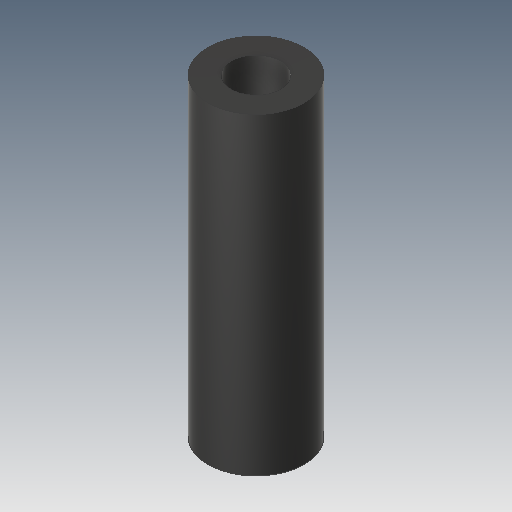
# Autodesk Inventor part: 20mm Nylon Stand Off
Saved by Autodesk Inventor 2019 (Build 230136000, 136)
## iProperties
Created: 2018-10-05
Part Number: 20mm Nylon Stand Off
Material: Acetal Resin, Black
Document SubType Name: Modeling
Designer: Ax
Density: 1.425 g/cm^3
Appearance: Smooth - Black
Mass: 0.637537 g
Surface Area: 6.40822 cm^2
Volume: 0.447394 cm^3
Author: Ax
Autodesk Inventor part; units mm, degrees
ref_plane "YZ Plane" through (0, 0, 0) normal (1, 0, 0) x (0, 1, 0)
ref_plane "XZ Plane" through (0, 0, 0) normal (0, 1, 0) x (-1, 0, 0)
ref_plane "XY Plane" through (0, 0, 0) normal (0, 0, 1) x (1, 0, 0)
sketch "Sketch1" plane through (0, 0, 0) normal (0, 1, 0) x (-1, 0, 0)
  circle A0 centre (0, 0) radius 3.1
  circle A1 centre (0, 0) radius 1.6
  dimension "d0" = 6.2
  dimension "d1" = 3.2
  constraints: 2 centre point, 2 coincident
  measures "d0" diameter of A0
  measures "d1" diameter of A1
extrude "Extrusion1" add sketch "Sketch1" along normal blind 20.2
body "Solid1"
